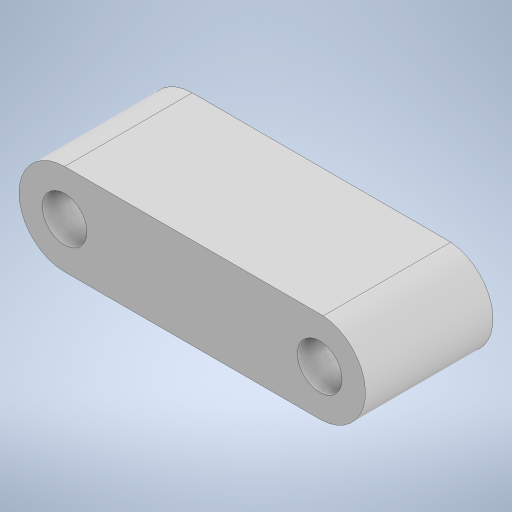
# Autodesk Inventor part: ArmMuscle
Saved by Autodesk Inventor 2023 (Build 270158000, 158)
## iProperties
Created: 2023-06-03
Part Number: ArmMuscle
Material: Ogólny
Document SubType Name: Modeling
Designer: Kamil
Density: 1 g/cm^3
Appearance: Domyślna
Author: Kamil
Autodesk Inventor part; units mm, degrees
ref_plane "YZ Plane" through (0, 0, 0) normal (1, 0, 0) x (0, 1, 0)
ref_plane "XZ Plane" through (0, 0, 0) normal (0, 1, 0) x (-1, 0, 0)
ref_plane "XY Plane" through (0, 0, 0) normal (0, 0, 1) x (1, 0, 0)
sketch "Szkic1" plane through (0, 0, 0) normal (0, 0, 1) x (1, 0, 0)
  line L0 (21.6558, 4.5742) -> (1.0948, 4.5742)
  circle A0 centre (1.3753, 0.9987) radius 3.5755
  circle A1 centre (1.3753, 0.9994) radius 1.7002
  line L1 (1.0948, -2.5758) -> (21.6558, -2.5758)
  circle A2 centre (21.3721, 1.0041) radius 3.5808
  circle A3 centre (21.3763, 0.9967) radius 1.6973
  point P0 (0, 0)
  point P1 (-2.1997, -2.5758)
  point P2 (1.3753, 4.5742)
  point P3 (1.2909, -2.5758)
  point P4 (21.4558, -2.5758)
  point P5 (21.6483, 4.5742)
  constraints: 4 centre point, 4 end point
extrude "Wyciągnięcie proste1" add sketch "Szkic1" along normal blind 10 contours A2 L0 | A2 L1 A0 L0 | A0 picked at (21.9206, 3.8831)
sketch "Szkic3" plane through (0, 0, 10) normal (0, 0, 1) x (1, 0, 0)
  circle A0 centre (1.3753, 0.9994) radius 1.7002 projected
  circle A1 centre (21.3763, 0.9967) radius 1.6973 projected
  circle A2 centre (1.3753, 0.9994) radius 1.75
  circle A3 centre (21.3763, 0.9967) radius 1.6973 projected
  circle A4 centre (21.3763, 0.9967) radius 1.75
  point P0 (0, 0)
  dimension "d13" = 3.5
  dimension "d14" = 3.5
  constraints: 2 centre point, 2 coincident
  measures "d13" diameter of A2
  measures "d14" diameter of A4
extrude "Wyciągnięcie proste3" cut sketch "Szkic3" against normal through all contours A0 | A1 | A2 | A4
